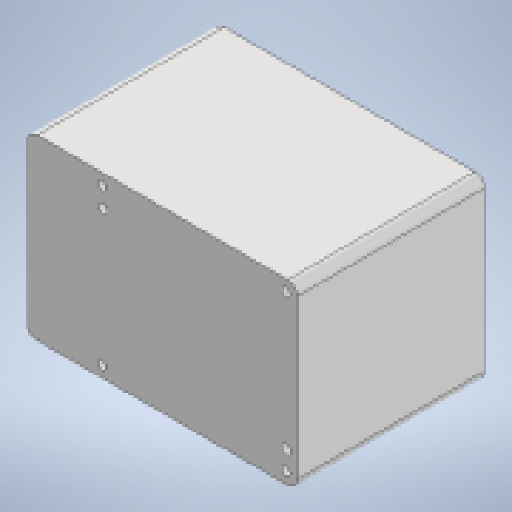
# Autodesk Inventor part: UPSboard
Saved by Autodesk Inventor 2025.1 (Build 291241000, 241)
## iProperties
Created: 2025-05-22
Part Number: UPSboard
Material: Generic
Document SubType Name: Modeling
Designer: User
Density: 1 g/cm^3
Appearance: Default
Author: User
Autodesk Inventor part; units mm, degrees
ref_plane "YZ Plane" through (0, 0, 0) normal (1, 0, 0) x (0, 1, 0)
ref_plane "XZ Plane" through (0, 0, 0) normal (0, 1, 0) x (-1, 0, 0)
ref_plane "XY Plane" through (0, 0, 0) normal (0, 0, 1) x (1, 0, 0)
sketch "Sketch1" plane through (0, 0, 0) normal (0, 0, 1) x (1, 0, 0)
  line L0 (-28, 61) -> (-28, 11) projected
  arc A0 (-28, 61) -> (-31, 64) centre (-31, 61) ccw projected
  line L1 (-110, 64) -> (-31, 64) projected
  arc A1 (-110, 64) -> (-113, 61) centre (-110, 61) ccw projected
  line L2 (-113, 11) -> (-113, 61) projected
  arc A2 (-113, 11) -> (-110, 8) centre (-110, 11) ccw projected
  line L3 (-31, 8) -> (-110, 8) projected
  arc A3 (-31, 8) -> (-28, 11) centre (-31, 11) ccw projected
  circle A4 centre (-89.5855, 11.5) radius 1.3645 projected
  circle A5 centre (-89.5855, 60.5) radius 1.3645 projected
  circle A6 centre (-31.5, 60.5) radius 1.3645 projected
  circle A7 centre (-31.5, 11.5) radius 1.3645 projected
  circle A8 centre (-31.4673, 17.5489) radius 1.5 projected
  circle A9 centre (-89.237, 54.3009) radius 1.5 projected
  point P0 (0, 0)
extrude "Extrusion1" add sketch "Sketch1" along normal blind 59
body "Solid1"
